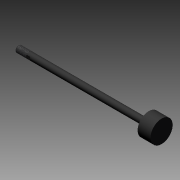
# Autodesk Inventor part: C-176-DP0_rod
Saved by Autodesk Inventor 2014 (Build 180170000, 170)
## iProperties
Created: 2014-01-18
Part Number: C-176-DP0_rod
Material: Steel
Catalog Web Link: www.cadenas.de
Description: Standard Air Cylinder_rod-Original Line - Standard Air Cylinders
Vendor: BIMBA
Document SubType Name: Standard Catalog Part
Designer: Andrew Toennies
Manufacturer: BIMBA
Density: 7.85 g/cm^3
Appearance: Steel
Mass: 372.975 g
Surface Area: 128.452 cm^2
Volume: 47.5128 cm^3
Category: PARTsolutions
Company: BIMBA
PSOL_IDENT_0: {$CADENAS_DATA\23d-libs\bimba\bimba\bimba_imperial\bimba_full_line\original_line_cylinders\standard_
PSOL_IDENT_1: air_cylinders\rod.prj},280 {VTYP=3D},{NB=C-176-DP0_rod},{LINA=C-176-DP0_rod},{NN=Standard Air Cylind
PSOL_IDENT_2: er_rod},{DATE=07.06.2013 09:21:38},{GEOMDATE=07.06.2013 09:21:38},{VERSION=},{LINEID=80},{LINESUBID=
PSOL_IDENT_3: -1},{WBVAR=STROKE,ACTING,MNT,DER,NR,BM,CO,M,EE,EEL,K,Q,Y,F,G,T,B,H,SER,SR,NT,W,E,HL,ST,STP,PRC,PB,CO
PSOL_IDENT_4: LOR1}  {NB=C-176-DP0_rod},{LINA=C-176-DP0_rod},{KT=DUMMY},{PN=C-176-DP},{DASH=-},{BORE=1.50000000},{
PSOL_IDENT_5: BOREPN=17},{STROKE=6.000},{STROKEALG=[0.001:50/0.001]},{STROKE1=6.000},{ACTING=D},{ACTINGALG= '' , '
PSOL_IDENT_6: Single Acting' , 'R' , 'Reverse Single Acting' , 'D' , 'Double Acting' },{ACTINGPN=D},{MNT=P},{MNTAL
PSOL_IDENT_7: G= '' , 'Front Nose Mounting' , 'P' , 'Rear Pivot Mounting' , 'X' , 'Universal Pivot Mounting or Dou
PSOL_IDENT_8: ble End Mounting' , 'BF' , 'Front Block Mounting' , 'BR' , 'Rear Block Mounting for Vertical Positio
PSOL_IDENT_9: ning' , 'BFT' , 'Front Block Trunnion Mounting' , 'BRT' , 'Rear Block Trunnion Mounting' },{TYPE=C-}
PSOL_IDENT_10: ,{MNTPN=P},{DER=},{DERALG= '' , 'N/A' },{NR=},{NRALG= '' , 'N/A' },{NRPN=},{BM=},{BMALG= '' , 'N/A'
PSOL_IDENT_11: },{BMPN=},{CO=},{COALG= '' , 'N/A' },{M=},{MALG= '', 'Without Magnet', 'M', 'With Magnet' },{EE=},{E
PSOL_IDENT_12: EL=0},{EEMAX=6},{EEALG= '', 'Without Extra Extension', 'EE', 'With Extra Extension' },{EELALG=0},{EE
PSOL_IDENT_13: PN=},{EEPN1=0.000},{K=},{KALG= '', 'Standard' , 'K' , 'Ports Rotated 90deg' },{KPN=},{Q=},{QALG= ''
PSOL_IDENT_14: , 'Without Side Ported Rear Head' , 'Q' , 'With Side Ported Rear Head' },{QPN=},{Y=},{YALG= '' , 'Wi
PSOL_IDENT_15: thout Pivot Bushing' , 'Y' , 'With Pivot Bushing' },{YPN=},{F=},{FALG= '', 'Standard', 'F', 'Molycoa
PSOL_IDENT_16: ted Body' },{FPN=},{G=},{GPN=},{T=},{TALG= '' , 'Standard' , 'N' , 'Low Temperature' , 'V' , 'High T
PSOL_IDENT_17: emperature' },{NPN=},{VPN=},{B=},{BALG= '', 'Without Bumper' , 'B' , 'With Bumper' },{BPN=},{H=},{HA
PSOL_IDENT_18: LG= '', 'N/A' },{HPN=},{SER=},{SERALG= '' , 'Without Spring Extend/Return' , 'JS' , 'With Spring Ret
PSOL_IDENT_19: urn' , 'JR' , 'With Spring Extend' },{SR=C},{SRALG= 'C' , 'Carbon Steel Rod' , 'SR' , '303 Stainless
PSOL_IDENT_20: Steel Rod' , '' , '303 Stainless Steel Rod1' },{SRPN=C},{SRCON=1},{NT=},{NTPN=},{W=},{WALG= '' , 'W
PSOL_IDENT_21: ithout Wiper' , 'W' , 'With Wiper' },{WPN=},{E=},{EALG= '' , 'Without Special Lube and Seals' , 'E'
PSOL_IDENT_22: , 'With Special Lube and Seals' },{EPN=},{HL=},{HLALG= '' , 'Wihout Low Pressure Hydraulic' , 'HL' ,
PSOL_IDENT_23: 'With Low Pressure Hydraulic' },{ST=},{STALG= '' , 'Without Switch Track' , 'T' , 'With Switch Trac
PSOL_IDENT_24: k' },{STP=},{STPALG= '' , 'N/A' },{STPN=},{PRC=},{PRCALG= '' , 'Without Piston Rod Clevis' , 'D-166-
PSOL_IDENT_25: 1' , 'With Piston Rod Clevis' },{PRCPN=},{PB=},{PBALG= '' , 'Without Pivot Bracket' , 'D-167' , 'Wit
PSOL_IDENT_26: h Pivot Bracket' },{PBPN=},{TLEN=7.3025},{TEXT=0.5},{SPACE=0.285714},{FRAC=45.3800},{RGCON=},{RGDACC
PSOL_IDENT_27: ON=R},{RHCON=P},{RHCONON=1},{RHACCON=R},{FNUTCON=0},{RNUTCON=0},{FNUTPN=},{RNUTPN=},{FNUTTRANS=0.000
PSOL_IDENT_28: 0},{RNUTTRANS=0.0000},{VHOLECON=0},{A1=1.8750},{A1N=1.3120},{A1P=1.8750},{A1B=2.3750},{A4=0.2525},{A
PSOL_IDENT_29: 4N=0.5000},{A4P=0.2525},{A5=0.0400},{A1H=1.75},{A1NH=0.6880},{A1PH=1.7500},{A1BH=1.3750},{A1SH=1.500
PSOL_IDENT_30: 0},{A2H=0.2500},{A2NH=0.2500},{LENGTH=4.3800},{LENGTH1=4.3800},{LENGTH2=4.4400},{MUL=6.0000},{MUL11=
PSOL_IDENT_31: 6.0000},{MUL22=16.1400},{MUL33=10.1400},{MUL2=6.0000},{MUL211=6.0000},{MUL222=2.6900},{MUL233=1.6900
PSOL_IDENT_32: },{SSS=12.0000},{RGLEN=1.6625},{RHLEN=1.1650},{SSS1=7.0000},{A13=1.3750},{THDLEN1=0.7500},{THD1=0.43
PSOL_IDENT_33: 75},{TAB=UNF},{THDLEN=0.7500},{THD=0.4375},{OD=1.5115},{RODL=9.7550},{PL=0.8800},{RODDIA=0.4370},{HE
PSOL_IDENT_34: X=0.4370},{RODTRANS=0.0000},{G1=0.0000},{ON=0},{G5=0.0000},{DERLEN=8.6250},{THOLE=0.2500},{WF=0.3800
PSOL_IDENT_35: },{BADD=0.0000},{MADD=0.0000},{NVADD=0.000},{JRADD=0.00000},{COLOR=0.00,0.00,0.00,0.00},{GROOVE=1},{
PSOL_IDENT_36: HOL=0},{D7=0.3775},{H1=1.6160},{D1=1.5565},{D1RH=1.5565},{D1P=1.5800},{D1B=1.5565},{D1N=1.5565},{D1N
PSOL_IDENT_37: RH=1.5565},{D1BRH=1.5800},{D1PRH=1.5565},{BOZO=0},{HADD=0.000},{COLOR1=0},{DEFL=0.0000},{HEXL=0.0000
PSOL_IDENT_38: },{SSADD=0.0000},{WFL=0.2500},{MOVE=0.2500},{PRCL2=0.75000},{PRCB=0.22000},{PRCTRANS=0.22000}
CNS_NN: Standard Air Cylinder_rod
CNS_NT: Standard
CNS_NB: C-176-DP0_rod
CNS_NBSYN: $PN.$COLOR1._rod
CNS_LINA: C-176-DP0_rod
CNS_PN: C-176-DP
CNS_DASH: -
CNS_BORE: 1.50000000
CNS_BOREPN: 17
CNS_STROKE: 6.000
CNS_STROKEALG: [0.001:50/0.001]
CNS_STROKE1: 6.000
CNS_ACTING: Double Acting
CNS_ACTINGALG: '' , 'Single Acting' , 'R' , 'Reverse Single Acting' , 'D' , 'Double Acting'
CNS_ACTINGPN: D
CNS_MNT: Rear Pivot Mounting
CNS_MNTALG: '' , 'Front Nose Mounting' , 'P' , 'Rear Pivot Mounting' , 'X' , 'Universal Pivot Mounting or Double End Mounting' , 'BF' , 'Front Block Mounting' , 'BR' , 'Rear Block Mounting for Vertical Positioning' , 'BFT' , 'Front Block Trunnion Mounting' , 'BRT' , 'Rear Block Trunnion Mounting'
CNS_TYPE: C-
CNS_MNTPN: P
CNS_DER: N/A
CNS_DERALG: '' , 'N/A'
CNS_NR: N/A
CNS_NRALG: '' , 'N/A'
CNS_BM: N/A
CNS_BMALG: '' , 'N/A'
CNS_CO: N/A
CNS_COALG: '' , 'N/A'
CNS_M: Without Magnet
CNS_MALG: '', 'Without Magnet', 'M', 'With Magnet'
CNS_EE: Without Extra Extension
CNS_EEL: 0
CNS_EEMAX: 6
CNS_EEALG: '', 'Without Extra Extension', 'EE', 'With Extra Extension'
CNS_EELALG: 0
CNS_EEPN1: 0.000
CNS_K: Standard
CNS_KALG: '', 'Standard' , 'K' , 'Ports Rotated 90deg'
CNS_Q: Without Side Ported Rear Head
CNS_QALG: '' , 'Without Side Ported Rear Head' , 'Q' , 'With Side Ported Rear Head'
CNS_Y: Without Pivot Bushing
CNS_YALG: '' , 'Without Pivot Bushing' , 'Y' , 'With Pivot Bushing'
CNS_F: Standard
CNS_FALG: '', 'Standard', 'F', 'Molycoated Body'
CNS_G: Without Magnalube Lubrication
CNS_T: Standard
CNS_TALG: '' , 'Standard' , 'N' , 'Low Temperature' , 'V' , 'High Temperature'
CNS_B: Without Bumper
CNS_BALG: '', 'Without Bumper' , 'B' , 'With Bumper'
CNS_H: N/A
CNS_HALG: '', 'N/A'
CNS_SER: Without Spring Extend/Return
CNS_SERALG: '' , 'Without Spring Extend/Return' , 'JS' , 'With Spring Return' , 'JR' , 'With Spring Extend'
CNS_SR: Carbon Steel Rod
CNS_SRALG: 'C' , 'Carbon Steel Rod' , 'SR' , '303 Stainless Steel Rod' , '' , '303 Stainless Steel Rod1'
CNS_SRPN: C
CNS_SRCON: 1
CNS_W: Without Wiper
CNS_WALG: '' , 'Without Wiper' , 'W' , 'With Wiper'
CNS_E: Without Special Lube and Seals
CNS_EALG: '' , 'Without Special Lube and Seals' , 'E' , 'With Special Lube and Seals'
CNS_HL: Wihout Low Pressure Hydraulic
CNS_HLALG: '' , 'Wihout Low Pressure Hydraulic' , 'HL' , 'With Low Pressure Hydraulic'
CNS_ST: Without Switch Track
CNS_STALG: '' , 'Without Switch Track' , 'T' , 'With Switch Track'
CNS_STP: N/A
CNS_STPALG: '' , 'N/A'
CNS_PRC: Without Piston Rod Clevis
CNS_PRCALG: '' , 'Without Piston Rod Clevis' , 'D-166-1' , 'With Piston Rod Clevis'
CNS_PB: Without Pivot Bracket
CNS_PBALG: '' , 'Without Pivot Bracket' , 'D-167' , 'With Pivot Bracket'
CNS_TLEN: 7.3025
CNS_TEXT: 0.500
CNS_SPACE: 0.286
CNS_FRAC: 45.3800
CNS_RGDACCON: R
CNS_RHCON: P
CNS_RHCONON: 1
CNS_RHACCON: R
CNS_FNUTCON: 0
CNS_RNUTCON: 0
CNS_FNUTTRANS: 0.0000
CNS_RNUTTRANS: 0.0000
CNS_VHOLECON: 0
CNS_A1: 1.8750
CNS_A1N: 1.3120
CNS_A1P: 1.8750
CNS_A1B: 2.3750
CNS_A4: 0.2525
CNS_A4N: 0.5000
CNS_A4P: 0.2525
CNS_A5: 0.0400
CNS_A1H: 1.750
CNS_A1NH: 0.6880
CNS_A1PH: 1.7500
CNS_A1BH: 1.3750
CNS_A1SH: 1.5000
CNS_A2H: 0.2500
CNS_A2NH: 0.2500
CNS_LENGTH: 4.3800
CNS_LENGTH1: 4.3800
CNS_LENGTH2: 4.4400
CNS_MUL: 6.0000
CNS_MUL11: 6.0000
CNS_MUL22: 16.1400
CNS_MUL33: 10.1400
CNS_MUL2: 6.0000
CNS_MUL211: 6.0000
CNS_MUL222: 2.6900
CNS_MUL233: 1.6900
CNS_SSS: 12.0000
CNS_RGLEN: 1.6625
CNS_RHLEN: 1.1650
CNS_SSS1: 7.0000
CNS_A13: 1.3750
CNS_THDLEN1: 0.7500
CNS_THD1: 0.4375
CNS_TAB: UNF
CNS_THDLEN: 0.7500
CNS_THD: 0.4375
CNS_OD: 1.5115
CNS_RODL: 9.7550
CNS_PL: 0.8800
CNS_RODDIA: 0.4370
CNS_HEX: 0.4370
CNS_RODTRANS: 0.0000
CNS_G1: 0.0000
CNS_ON: 0
CNS_G5: 0.0000
CNS_DERLEN: 8.6250
CNS_THOLE: 0.2500
CNS_WF: 0.3800
CNS_BADD: 0.0000
CNS_MADD: 0.0000
CNS_NVADD: 0.000
CNS_JRADD: 0.00000
CNS_COLOR: 0.00,0.00,0.00,0.00
CNS_GROOVE: 1
CNS_HOL: 0
CNS_D7: 0.3775
CNS_H1: 1.6160
CNS_D1: 1.5565
CNS_D1RH: 1.5565
CNS_D1P: 1.5800
CNS_D1B: 1.5565
CNS_D1N: 1.5565
CNS_D1NRH: 1.5565
CNS_D1BRH: 1.5800
CNS_D1PRH: 1.5565
CNS_BOZO: 0
CNS_HADD: 0.000
CNS_COLOR1: 0
CNS_DEFL: 0.0000
CNS_HEXL: 0.0000
CNS_SSADD: 0.0000
CNS_WFL: 0.2500
CNS_MOVE: 0.2500
CNS_PRCL2: 0.75000
CNS_PRCB: 0.22000
CNS_PRCTRANS: 0.22000
SUPPLIER: BIMBA
ARTICLENO: C-176-DP0_rod
BOMINFO: C-176-DP0_rod
CREATOR: CADENAS GmbH
Title: C-176-DP0_rod
Author: Cadenas PARTsolutions
Comments: Original Line - Standard Air Cylinders
Autodesk Inventor part; units mm, degrees
sketch "Sketch_1" plane through (0, 0, 0) normal (0, 0, 1) x (1, 0, 0)
  line L0 (222.377, 0) -> (-6.35, 0)
  line L1 (-6.35, 0) -> (-6.35, 5.5499)
  line L2 (-6.35, 5.5499) -> (200.025, 5.5499)
  line L3 (200.025, 5.5499) -> (200.025, 19.1453)
  line L4 (200.025, 19.1453) -> (222.377, 19.1453)
  line L5 (222.377, 19.1453) -> (222.377, 0)
  line L6 (222.377, 0) -> (-6.35, 0)
  constraints: 14 end point
revolve "Revolution1" add sketch "Sketch_1" angle 360 about axis through (222.377, 0, 0) along (1, 0, 0)
sketch "Sketch_3" plane through (0, 0, 0) normal (0, 0, 1) x (1, 0, 0)
  line L0 (-6.35, 0) -> (-25.4, 0)
  line L1 (-25.4, 0) -> (-25.4, 4.8006)
  line L2 (-25.4, 4.8006) -> (-24.6443, 5.5563)
  line L3 (-24.6443, 5.5563) -> (-6.35, 5.5563)
  line L4 (-6.35, 5.5563) -> (-6.35, 0)
  line L5 (-6.35, 0) -> (-25.4, 0)
  constraints: 12 end point
revolve "Revolution2" add sketch "Sketch_3" angle 360 about axis through (-6.35, 0, 0) along (1, 0, 0)
thread "Thread1" size "7/16-20 UNF" class "2A" standard "ANSI Unified Screw Threads" full length
sketch "Sketch_10" plane through (-6.35, 0, 0) normal (1, 0, 0) x (0, 0, -1)
  line L0 (-11.0998, 11.0998) -> (-11.0998, -11.0998)
  line L1 (-11.0998, -11.0998) -> (11.0998, -11.0998)
  line L2 (11.0998, -11.0998) -> (11.0998, 11.0998)
  line L3 (11.0998, 11.0998) -> (-11.0998, 11.0998)
  line L4 (-4.826, 5.5499) -> (-4.826, -5.5499)
  line L5 (-4.826, -5.5499) -> (4.826, -5.5499)
  line L6 (4.826, -5.5499) -> (4.826, 5.5499)
  line L7 (4.826, 5.5499) -> (-4.826, 5.5499)
  constraints: 16 end point
extrude "Extrusion1" cut sketch "Sketch_10" along normal blind 6.35
ref_plane "dia1_XY" through (-6.35, 5.5499, 0) normal (1, 0, 0) x (0, 0, -1)
ref_plane "dia1_YZ" through (-6.35, 5.5499, 0) normal (0, 0, -1) x (0, 1, 0)
ref_plane "dia1_ZX" through (-6.35, 5.5499, 0) normal (0, 1, 0) x (1, 0, 0)
ref_plane "dia12_XY" through (0, 0, 19.7675) normal (1, 0, 0) x (0, 0, -1)
ref_plane "dia12_YZ" through (0, 0, 19.7675) normal (0, 0, -1) x (0, 1, 0)
ref_plane "dia12_ZX" through (0, 0, 19.7675) normal (0, 1, 0) x (1, 0, 0)
ref_plane "dia2_XY" through (-6.35, -5.5499, 0) normal (1, 0, 0) x (0, 0, -1)
ref_plane "dia2_YZ" through (-6.35, -5.5499, 0) normal (0, 0, -1) x (0, 1, 0)
ref_plane "dia2_ZX" through (-6.35, -5.5499, 0) normal (0, 1, 0) x (1, 0, 0)
ref_plane "dia22_XY" through (0, 0, -19.7675) normal (1, 0, 0) x (0, 0, -1)
ref_plane "dia22_YZ" through (0, 0, -19.7675) normal (0, 0, -1) x (0, 1, 0)
ref_plane "dia22_ZX" through (0, 0, -19.7675) normal (0, 1, 0) x (1, 0, 0)
ref_plane "rl1_XY" through (-25.4, 0, 0) normal (1, 0, 0) x (0, 0, -1)
ref_plane "rl1_YZ" through (-25.4, 0, 0) normal (0, 0, -1) x (0, 1, 0)
ref_plane "rl1_ZX" through (-25.4, 0, 0) normal (0, 1, 0) x (1, 0, 0)
ref_plane "rl2_XY" through (-6.35, 0, 0) normal (1, 0, 0) x (0, 0, -1)
ref_plane "rl2_YZ" through (-6.35, 0, 0) normal (0, 0, -1) x (0, 1, 0)
ref_plane "rl2_ZX" through (-6.35, 0, 0) normal (0, 1, 0) x (1, 0, 0)
ref_plane "rod_cp_XY" through (0, 0, 0) normal (1, 0, 0) x (0, 0, -1)
ref_plane "rod_cp_YZ" through (0, 0, 0) normal (0, 0, -1) x (0, 1, 0)
ref_plane "rod_cp_ZX" through (0, 0, 0) normal (0, 1, 0) x (1, 0, 0)
ref_plane "thd1_XY" through (-25.4, 5.5563, 0) normal (1, 0, 0) x (0, 0, -1)
ref_plane "thd1_YZ" through (-25.4, 5.5563, 0) normal (0, 0, -1) x (0, 1, 0)
ref_plane "thd1_ZX" through (-25.4, 5.5563, 0) normal (0, 1, 0) x (1, 0, 0)
ref_plane "thd2_XY" through (-25.4, -5.5563, 0) normal (1, 0, 0) x (0, 0, -1)
ref_plane "thd2_YZ" through (-25.4, -5.5563, 0) normal (0, 0, -1) x (0, 1, 0)
ref_plane "thd2_ZX" through (-25.4, -5.5563, 0) normal (0, 1, 0) x (1, 0, 0)
ref_plane "to_rod_clevis_XY" through (-30.988, 0, 0) normal (1, 0, 0) x (0, 0, -1)
ref_plane "to_rod_clevis_YZ" through (-30.988, 0, 0) normal (0, 0, -1) x (0, 1, 0)
ref_plane "to_rod_clevis_ZX" through (-30.988, 0, 0) normal (0, 1, 0) x (1, 0, 0)
ref_plane "wf1_XY" through (-6.35, 0, 0) normal (1, 0, 0) x (0, 0, -1)
ref_plane "wf1_YZ" through (-6.35, 0, 0) normal (0, 0, -1) x (0, 1, 0)
ref_plane "wf1_ZX" through (-6.35, 0, 0) normal (0, 1, 0) x (1, 0, 0)
ref_plane "wf2_XY" through (0, 0, 0) normal (1, 0, 0) x (0, 0, -1)
ref_plane "wf2_YZ" through (0, 0, 0) normal (0, 0, -1) x (0, 1, 0)
ref_plane "wf2_ZX" through (0, 0, 0) normal (0, 1, 0) x (1, 0, 0)
ref_plane "wfw1_XY" through (-6.35, 0, -4.826) normal (0, 1, 0) x (1, 0, 0)
ref_plane "wfw1_YZ" through (-6.35, 0, -4.826) normal (1, 0, 0) x (0, 0, -1)
ref_plane "wfw1_ZX" through (-6.35, 0, -4.826) normal (0, 0, -1) x (0, 1, 0)
ref_plane "wfw2_XY" through (-6.35, 0, 4.826) normal (0, 1, 0) x (1, 0, 0)
ref_plane "wfw2_YZ" through (-6.35, 0, 4.826) normal (1, 0, 0) x (0, 0, -1)
ref_plane "wfw2_ZX" through (-6.35, 0, 4.826) normal (0, 0, -1) x (0, 1, 0)
body "Solid1"
